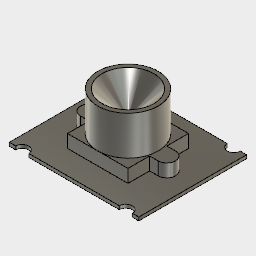
Polariser Mount v5 (Autodesk Fusion 360 archive; units mm, degrees)
design "camera hbv-1517"
Autodesk Fusion 360 part; units mm, degrees
sketch "Sketch1" plane through (0, 0, 0) normal (0, 0, 1) x (1, 0, 0)
  line L0 (15, 12.5) -> (-15, -12.5) construction
  line L1 (-15, 12.5) -> (15, -12.5) construction
  line L2 (-15, 12.5) -> (-15, 10.9975)
  line L3 (-5.5, 0) -> (4.5, 0) construction
  line L4 (0, 4.5) -> (0, -5.5) construction
  line L5 (-15, 7.9975) -> (-15, -7.9975)
  line L6 (-15, -10.9975) -> (-15, -12.5)
  line L7 (15, -12.5) -> (15, -10.9975)
  line L8 (15, -7.9975) -> (15, 7.9975)
  line L9 (15, 10.9975) -> (15, 12.5)
  line L10 (-15, -10.9975) -> (-15, -7.9975)
  line L11 (-15, 7.9975) -> (-15, 10.9975)
  line L12 (15, -10.9975) -> (15, -7.9975)
  line L13 (15, 7.9975) -> (15, 10.9975)
  arc A0 (-13.5, 12.5) -> (-10.5, 12.5) centre (-12, 12.5) ccw
  line L14 (-13.5, 12.5) -> (-15, 12.5)
  line L15 (-15, -12.5) -> (-13.5, -12.5)
  arc A1 (10.5, 12.5) -> (13.5, 12.5) centre (12, 12.5) ccw
  arc A2 (-10.5, -12.5) -> (-13.5, -12.5) centre (-12, -12.5) ccw
  arc A3 (13.5, -12.5) -> (10.5, -12.5) centre (12, -12.5) ccw
  line L16 (15, 12.5) -> (13.5, 12.5)
  line L17 (-10.5, 12.5) -> (10.5, 12.5)
  line L18 (-10.5, -12.5) -> (10.5, -12.5)
  line L19 (13.5, -12.5) -> (15, -12.5)
  dimension "d1" = 30
  dimension "d2" = 25
  dimension "d23" = 30
  dimension "d25" = 1.5
  dimension "d27" = 12
  measures "d1" distance of L0.end L1.end
  measures "d2" distance of L1.start L0.end
  measures "d23" distance of L5 L8
  measures "d25" radius of A0
  measures "d27" distance of L4.start A0.centre
extrude "Extrude1" add sketch "Sketch1" along normal blind 0.8
sketch "Sketch2" plane through (0, 0, 0.8) normal (0, 0, 1) x (-1, 0, 0)
  line L0 (-15, 12.5) -> (-15, -12.5)
  line L1 (15, -12.5) -> (15, 12.5)
  line L2 (15, 12.5) -> (13.5, 12.5)
  line L3 (-7, -7) -> (7, -7)
  line L4 (7, 7) -> (-7, 7)
  line L5 (-7, -7) -> (7, 7) construction
  line L6 (7, -7) -> (-7, 7) construction
  arc A0 (-8.9996, 2) -> (-9.0004, -2) centre (-9, 0) ccw
  arc A1 (9, -2) -> (9, 2) centre (9, 0) ccw
  line L7 (9, -2) -> (7, -2)
  line L8 (9, 2) -> (7, 2)
  line L9 (-9.0004, -2) -> (-7, -2)
  line L10 (-8.9996, 2) -> (-7, 1.9996)
  line L11 (-7, 7) -> (-7, 1.9996)
  line L12 (-7, -2) -> (-7, -7)
  line L13 (7, -7) -> (7, -2)
  line L14 (7, 2) -> (7, 7)
  arc A2 (13.5, -12.5) -> (10.5, -12.5) centre (12, -12.5) ccw
  line L15 (13.5, -12.5) -> (15, -12.5)
  line L16 (10.5, 12.5) -> (-10.5, 12.5)
  arc A3 (-13.5, 12.5) -> (-10.5, 12.5) centre (-12, 12.5) ccw
  line L17 (-13.5, 12.5) -> (-15, 12.5)
  line L18 (-15, -12.5) -> (-13.5, -12.5)
  arc A4 (-10.5, -12.5) -> (-13.5, -12.5) centre (-12, -12.5) ccw
  line L19 (-10.5, -12.5) -> (10.5, -12.5)
  arc A5 (10.5, 12.5) -> (13.5, 12.5) centre (12, 12.5) ccw
  dimension "d5" = 14
  dimension "d6" = 14
  measures "d5" distance of L4.start L4.end
  measures "d6" distance of L3.end L4.start
extrude "Extrude2" add sketch "Sketch2" along normal blind 3 contours L3 L4 A0 A1 L7 L8 L9 L10 L11 L12 L13 L14
sketch "Sketch3" plane through (0, 0, 3.8) normal (0, 0, 1) x (-1, 0, 0)
  arc A0 (9, -2) -> (9, 2) centre (9, 0) ccw
  line L0 (9, 2) -> (7, 2)
  line L1 (7, 2) -> (7, 7)
  line L2 (7, 7) -> (-7, 7)
  line L3 (-7, 7) -> (-7, 1.9996)
  line L4 (-7, 1.9996) -> (-8.9996, 2)
  arc A1 (-8.9996, 2) -> (-9.0004, -2) centre (-9, 0) ccw
  line L5 (-9.0004, -2) -> (-7, -2)
  line L6 (-7, -2) -> (-7, -7)
  line L7 (-7, -7) -> (7, -7)
  line L8 (7, -7) -> (7, -2)
  line L9 (7, -2) -> (9, -2)
  circle A2 centre (0, 0) radius 7
  dimension "d9" = 14
  measures "d9" diameter of A2
extrude "Extrude3" add sketch "Sketch3" along normal blind 9 contours A2
sketch "Sketch4" plane through (0, 0, 12.8) normal (0, 0, 1) x (-1, 0, 0)
  circle A0 centre (0, 0) radius 7
  circle A1 centre (0, 0) radius 1
extrude "Extrude4" cut sketch "Sketch4" against normal blind 6 contours A1
chamfer "Chamfer1" distance 5 angle 45 1 edges at (0.9323, -0.3616, 12.8)
sketch "Sketch5" plane through (0, 0, 0) normal (0, 0, -1) x (1, 0, 0)
  line L0 (15, -12.5) -> (15, 12.5)
  line L1 (-13.5, 12.5) -> (-15, 12.5)
  line L2 (-15, 12.5) -> (-15, -12.5)
  line L3 (-15, -12.5) -> (-13.5, -12.5)
  line L4 (5.4544, -12.5) -> (-1.5456, -12.5)
  line L5 (-1.5456, -12.5) -> (-1.5456, -8)
  line L6 (-1.5456, -8) -> (5.4544, -8)
  line L7 (5.4544, -8) -> (5.4544, -12.5)
  arc A0 (-10.5, -12.5) -> (-13.5, -12.5) centre (-12, -12.5) ccw
  line L8 (10.5, 12.5) -> (-10.5, 12.5)
  arc A1 (-13.5, 12.5) -> (-10.5, 12.5) centre (-12, 12.5) ccw
  line L9 (-10.5, -12.5) -> (10.5, -12.5)
  arc A2 (13.5, -12.5) -> (10.5, -12.5) centre (12, -12.5) ccw
  line L10 (13.5, -12.5) -> (15, -12.5)
  line L11 (15, 12.5) -> (13.5, 12.5)
  arc A3 (10.5, 12.5) -> (13.5, 12.5) centre (12, 12.5) ccw
  dimension "d15" = 7
  dimension "d16" = 4.5
  measures "d15" distance of L4.start L4.end
  measures "d16" distance of L4.start L6.end
extrude "Extrude5" add sketch "Sketch5" along normal blind 3 contours L4 L5 L6 L7 L9
sketch "Sketch6" plane through (0, 12.5, 0) normal (0, 1, 0) x (-1, 0, 0)
  line L0 (1.5456, 0) -> (10.5, 0)
  line L1 (-5.4544, 0) -> (-5.4544, -3)
  line L2 (-5.4544, -3) -> (1.5456, -3)
  line L3 (1.5456, -3) -> (1.5456, 0)
  line L4 (10.5, 0.8) -> (-10.5, 0.8)
  line L5 (-5, -2.5) -> (1, -2.5)
  line L6 (1, -2.5) -> (1, -0.5)
  line L7 (1, -0.5) -> (-5, -0.5)
  line L8 (-5, -0.5) -> (-5, -2.5)
  line L9 (10.5, 0) -> (10.5, 0.8)
  line L10 (-10.5, 0.8) -> (-10.5, 0)
  line L11 (-10.5, 0) -> (-5.4544, 0)
extrude "Extrude6" cut sketch "Sketch6" against normal blind 3 contours L5 L6 L7 L8
